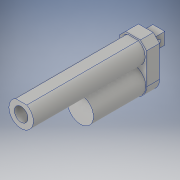
# Autodesk Inventor part: actuator_base
Saved by Autodesk Inventor 2019.4 (Build 234330000, 330)
## iProperties
Created: 2020-10-05
Part Number: actuator_base
Material: Aluminum 6061
Document SubType Name: Modeling
Designer: deanv
Density: 2.7 g/cm^3
Appearance: Aluminum - Flat
Author: deanv
Autodesk Inventor part; units mm, degrees
ref_plane "YZ Plane" through (0, 0, 0) normal (1, 0, 0) x (0, 1, 0)
ref_plane "XZ Plane" through (0, 0, 0) normal (0, 1, 0) x (-1, 0, 0)
ref_plane "XY Plane" through (0, 0, 0) normal (0, 0, 1) x (1, 0, 0)
sketch "Sketch1" plane through (0, 0, 0) normal (0, 0, 1) x (1, 0, 0)
  line L0 (-20, -37.4) -> (20, -37.4) construction
  line L1 (20, -37.4) -> (20, 37.4) construction
  line L2 (20, 37.4) -> (-20, 37.4) construction
  line L3 (-20, 37.4) -> (-20, -37.4) construction
  line L4 (-20, -37.4) -> (20, 37.4) construction
  line L5 (20, -37.4) -> (-20, 37.4) construction
  line L6 (0, 37.4) -> (0, -37.4) construction
  line L7 (-20, 0) -> (20, 0) construction
  circle A0 centre (0, -17.4) radius 19
  line L8 (8.75, 10.75) -> (-8.75, 10.75)
  line L9 (-8.75, 10.75) -> (-8.75, 28.25)
  line L10 (-8.75, 28.25) -> (8.75, 28.25)
  line L11 (8.75, 28.25) -> (8.75, 10.75)
  line L12 (8.75, 10.75) -> (-8.75, 28.25) construction
  line L13 (-8.75, 10.75) -> (8.75, 28.25) construction
  line L14 (20, 1.6) -> (-20, 1.6) construction
  line L15 (-20, 37.4) -> (-10.85, 37.4) construction
  line L16 (-10.85, 37.4) -> (-10.85, 28.25) construction
  line L17 (-10.85, 28.25) -> (-20, 28.25) construction
  line L18 (-20, 28.25) -> (-20, 37.4) construction
  line L19 (20, 37.4) -> (10.85, 37.4) construction
  line L20 (10.85, 37.4) -> (10.85, 28.25) construction
  line L21 (10.85, 28.25) -> (20, 28.25) construction
  line L22 (20, 28.25) -> (20, 37.4) construction
  line L23 (-10.85, 37.4) -> (-20, 28.25)
  line L24 (-20, -17.4) -> (20, -17.4) construction
  arc A1 (-20, -17.4) -> (20, -17.4) centre (0, -17.4) ccw
  line L25 (-20, 28.25) -> (-20, -17.4)
  line L26 (20, -17.4) -> (20, 28.25)
  line L27 (20, 28.25) -> (10.85, 37.4)
  line L28 (10.85, 37.4) -> (-10.85, 37.4)
  circle A2 centre (0, 19.5) radius 17.9 construction
  circle A3 centre (0, 19.5) radius 10
  line L29 (-8.2219, 35.4) -> (8.2219, 35.4)
  arc A4 (-8.2219, 35.4) -> (8.2219, 35.4) centre (0, 19.5) ccw
  point P0 (0, 0)
  point P1 (0, 1.6)
  point P2 (-10.85, 33.7368)
  point P3 (10.85, 33.7368)
  dimension "d2" = 38
  dimension "d0" = 40
  dimension "d1" = 74.8
  dimension "d3" = 20
  dimension "d4" = 17.5
  dimension "d5" = 17.5
  dimension "d6" = 35.8
  dimension "d7" = 9.15
  dimension "d8" = 9.15
  dimension "d9" = 9.15
  dimension "d10" = 9.15
  dimension "d11" = 9.15
  dimension "d12" = 45.65
  dimension "d21" = 20
  dimension "d22" = 2
  constraints: 60 end point, 10 point on circle, 9 midpoint, 9 parallel, 9 point on line, 7 perpendicular, 5 horizontal, 4 centre point, 2 concentric, 1 coincident, 1 collinear, 1 vertical alignment, 2 other
  measures "d0" distance of L2.end L1.end
  measures "d1" distance of L1.end L0.end
  measures "d3" distance from line of L0 point (0, -17.4)
  measures "d4" distance of L9.end L10.end
  measures "d5" distance of L8.end L9.end
  measures "d6" distance between parallel lines of L2 L14
  measures "d7" distance between parallel lines of L2 L10
  measures "d8" distance of L15.end L16.end
  measures "d9" distance between parallel lines of L16 L3
  measures "d10" distance between parallel lines of L1 L20
  measures "d11" distance between parallel lines of L19 L21
  measures "d12" distance between parallel lines of L24 L21
  measures "d21" diameter of A3
  measures "d22" distance between parallel lines of L2 L29
extrude "Extrusion1" add sketch "Sketch1" along normal blind 95.7 contours A0
extrude "Extrusion2" add sketch "Sketch1" against normal blind 19 contours L8 A3 L11 | L8 A3 L9 L10 L11 | L8 L9 A3 | A3 L10 L11 | L9 L10 A3
extrude "Extrusion3" add sketch "Sketch1" along normal blind 19 contours A4 L29 | A3 L8 | L11 A3 | A3 L9 | L10 A3 | L28 L27 L26 A1 L25 L23
extrude "Extrusion5" add sketch "Sketch1" along normal blind 182.5 contours A4 L29 | L8 A3 L11 | A3 L8 | L8 A3 L9 L10 L11 | L11 A3 | L8 L9 A3 | A3 L10 L11 | A3 L9 | L10 A3 | L9 L10 A3
extrude "Extrusion6" cut sketch "Sketch1" along normal blind 182.5 contours A3 L8 | L8 A3 L9 L10 L11 | L11 A3 | A3 L9 | L10 A3
extrude "Extrusion7" add sketch "Sketch1" along normal blind 32.5 contours A3 L8 | L8 A3 L9 L10 L11 | L11 A3 | A3 L9 | L10 A3
sketch "Sketch2" plane through (-8.75, 10.75, 0) normal (-1, 0, 0) x (0, 0, 1)
  line L0 (0, 26.65) -> (0, 17.5) construction
  line L1 (0, 0) -> (-19, 0) construction
  line L2 (0, 17.5) -> (-10, 17.5) construction
  line L3 (-10, 17.5) -> (-10, 0) construction
  line L4 (-10, 0) -> (0, 0) construction
  line L5 (0, 0) -> (0, 17.5) construction
  point P0 (0, -10.75)
  point P1 (-10, 8.75)
  dimension "d29" = 10
  constraints: 8 end point, 2 parallel, 1 horizontal, 1 midpoint, 1 perpendicular, 1 point on line
  measures "d29" distance of L4.end L3.end
hole "Hole1" at (-8.75, 19.5, -10) direction (1, 0, 0) diameter 6 end through all both
equation "\"d5\" = d4"
equation "\"d7\" = 0.5 * d6 - 0.5 * d4"
equation "\"d9\" = d8"
equation "\"d10\" = d9"
equation "\"d11\" = d10"
body "Solid1"
